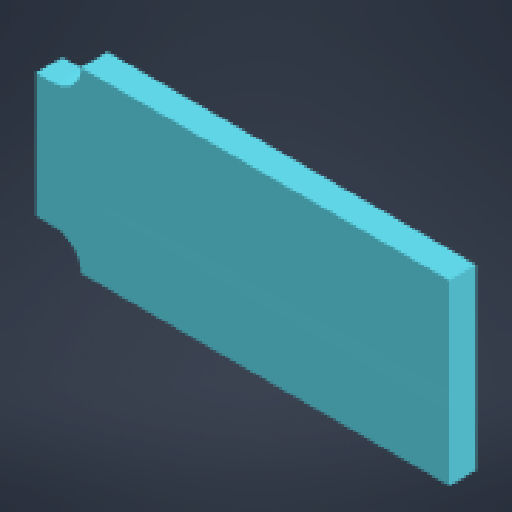
# Autodesk Inventor part: tibea_reinforcement_steel
Saved by Autodesk Inventor 2026 (Build 300175000, 175)
## iProperties
Created: 2026-05-02
Part Number: tibea_reinforcement_steel
Material: Сталь
Document SubType Name: Modeling
Designer: user
Density: 7.85 g/cm^3
Appearance: Серо-синий
Mass: 20.8338 g
Surface Area: 21.564 cm^2
Volume: 2.65399 cm^3
Author: user
Autodesk Inventor part; units mm, degrees
ref_plane "YZ Plane" through (0, 0, 0) normal (1, 0, 0) x (0, 1, 0)
ref_plane "XZ Plane" through (0, 0, 0) normal (0, 1, 0) x (-1, 0, 0)
ref_plane "XY Plane" through (0, 0, 0) normal (0, 0, 1) x (1, 0, 0)
sketch "Эскиз3" plane through (0, 0, 0) normal (0, 0, 1) x (1, 0, 0)
  line L0 (3, 0) -> (44, 0)
  line L1 (44, 19.8) -> (3, 19.8)
  arc A0 (0, 16.8) -> (3, 19.8) centre (0, 19.8) ccw
  arc A1 (3, 0) -> (0, 3) centre (0, 0) ccw
  line L2 (-9.5212, 9.95) -> (-2, 9.95) construction
  line L3 (0, 16.8) -> (-2, 16.8)
  line L4 (-2, 16.8) -> (-2, 3)
  line L5 (-2, 3) -> (0, 3)
  line L6 (44, 19.8) -> (44, 0)
  point P0 (36.5732, 9.95)
  dimension "d10" = 6
  dimension "d11" = 19.8
  dimension "d13" = 2
  dimension "d14" = 46
  constraints: 14 end point, 4 horizontal alignment, 4 point on circle, 3 horizontal, 3 vertical alignment, 2 centre point, 2 point on line, 1 coincident, 1 equal radius, 1 parallel, 1 perpendicular, 1 vertical
  measures "d10" diameter of A0
  measures "d11" distance between parallel lines of L0 L1
  measures "d13" distance of L3.start L3.end
  measures "d14" distance from line of L4 L0.end
extrude "Выдавливание3" add sketch "Эскиз3" along normal blind 3
equation "\"d11\" = width_profile_tibea - 2 * tolerance_plazma"
equation "\"d6\" = thickness_steel"
equation "\"tolerance_plazma\" = 0.1"
equation "\"thickness_steel\" = 3"
equation "\"d_main_screw_holes\" = 6.1"
equation "\"thickness_profile_tibea\" = 3"
equation "\"hight_shaft_shift\" = 37"
equation "\"thickness_profile_femur\" = 3"
equation "\"width_shaft_shift\" = 35"
equation "\"width_flattened_surface\" = 12"
equation "\"width_profile_tibea\" = 20"
